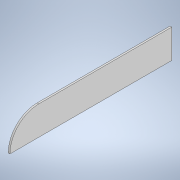
# Autodesk Inventor part: Part7
Saved by Autodesk Inventor 2022 (Build 260153000, 153)
## iProperties
Created: 2021-12-09
Part Number: Part7
Material: Generic
Document SubType Name: Modeling
Designer: keemi
Density: 1 g/cm^3
Appearance: Default
Author: keemi
Autodesk Inventor part; units mm, degrees
ref_plane "YZ Plane" through (0, 0, 0) normal (1, 0, 0) x (0, 1, 0)
ref_plane "XZ Plane" through (0, 0, 0) normal (0, 1, 0) x (-1, 0, 0)
ref_plane "XY Plane" through (0, 0, 0) normal (0, 0, 1) x (1, 0, 0)
sketch "Sketch1" plane through (0, 0, 0) normal (1, 0, 0) x (0, 1, 0)
  line L0 (0, 0) -> (0, -280)
  line L1 (0, -280) -> (50, -280)
  line L2 (50, -280) -> (50, -50)
  line L3 (0, 0) -> (0, 0)
  arc A0 (50, -50) -> (0, 0) centre (0, -50) ccw
  dimension "d0" = 280
  dimension "d1" = 50
  dimension "d2" = 90
  dimension "d3" = 50
  constraints: 8 end point, 3 perpendicular, 2 point on circle, 2 tangent, 1 centre point, 1 vertical
  measures "d0" distance of L0.start L0.end
  measures "d1" distance of L0.end L1.end
  measures "d2" angle of L1 L0
  measures "d3" radius of A0
extrude "Extrusion1" add sketch "Sketch1" along normal blind 3
body "Solid1"
